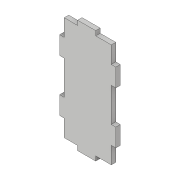
# Autodesk Inventor part: costat2
Saved by Autodesk Inventor 2019 (Build 230136000, 136)
## iProperties
Created: 2018-09-21
Part Number: costat2
Material: Genérico
Document SubType Name: Modeling
Designer: lmacia
Density: 1 g/cm^3
Appearance: Valor por defecto
Author: lmacia
Autodesk Inventor part; units mm, degrees
ref_plane "YZ Plane" through (0, 0, 0) normal (1, 0, 0) x (0, 1, 0)
ref_plane "XZ Plane" through (0, 0, 0) normal (0, 1, 0) x (-1, 0, 0)
ref_plane "XY Plane" through (0, 0, 0) normal (0, 0, 1) x (1, 0, 0)
sketch "Boceto1" plane through (0, 0, 0) normal (0, 0, 1) x (-1, 0, 0)
  line L0 (-15.8165, -11.3864) -> (-18.8665, -11.3864)
  line L1 (-18.8665, -11.3864) -> (-18.8665, -23.5865)
  line L2 (-18.8665, -23.5865) -> (-15.8165, -23.5865)
  line L3 (-15.8165, -23.5865) -> (-15.8165, -34.9987)
  line L4 (-15.8165, -34.9987) -> (-5.2939, -34.9987)
  line L5 (-5.2939, -34.9987) -> (-5.2939, -38.0488)
  line L6 (-5.2939, -38.0488) -> (6.9062, -38.0488)
  line L7 (6.9062, -38.0488) -> (6.9062, -34.9987)
  line L8 (6.9062, -34.9987) -> (15.9038, -34.9987)
  line L9 (15.9038, -34.9987) -> (15.9038, -23.5874)
  line L10 (15.9038, -23.5874) -> (18.9539, -23.5865)
  line L11 (18.9539, -23.5865) -> (18.9539, -11.3864)
  line L12 (18.9539, -11.3864) -> (15.9038, -11.3864)
  line L13 (15.9038, -11.3864) -> (15.9038, 11.438)
  line L14 (15.9038, 11.438) -> (18.9539, 11.438)
  line L15 (18.9539, 11.438) -> (18.9539, 23.6381)
  line L16 (18.9539, 23.6381) -> (15.9038, 23.6381)
  line L17 (15.9038, 23.6381) -> (15.9038, 28.9502)
  line L18 (15.9038, 28.9502) -> (15.9038, 35.0503)
  line L19 (15.9038, 35.0503) -> (6.9062, 35.0503)
  line L20 (6.9062, 35.0503) -> (6.9062, 38.1003)
  line L21 (6.9062, 38.1003) -> (-5.2939, 38.1003)
  line L22 (-5.2939, 38.1003) -> (-5.2939, 35.0503)
  line L23 (-5.2939, 35.0503) -> (-14.2915, 35.0503)
  line L24 (-14.2915, 35.0503) -> (-14.7998, 35.0503)
  line L25 (-14.7998, 35.0503) -> (-15.8165, 35.0503)
  line L26 (-15.8165, 35.0503) -> (-15.8165, 23.6381)
  line L27 (-15.8165, 23.6381) -> (-18.8665, 23.6381)
  line L28 (-18.8665, 23.6381) -> (-18.8665, 11.438)
  line L29 (-18.8665, 11.438) -> (-15.8165, 11.438)
  line L30 (-15.8165, 11.438) -> (-15.8165, -11.3864)
  dimension "d2" = 76.149
  dimension "d3" = 37.82
  constraints: 62 end point
  measures "d2" distance between parallel lines of L21 L6
extrude "Extrusión1" add sketch "Boceto1" along normal blind 3
